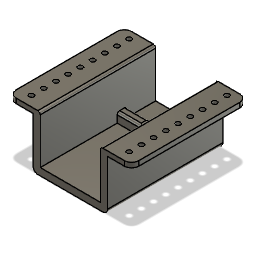
Motor mount (Autodesk Fusion 360 design; units mm, degrees)
Autodesk Fusion 360 part; units mm, degrees
sketch "Sketch1" plane through (0, 0, 0) normal (0, 1, 0) x (1, 0, 0)
  line L0 (0, 0) -> (12.5, 0)
  line L1 (12.5, 0) -> (12.5, 24)
  line L2 (12.5, 24) -> (0, 24)
  line L3 (0, 24) -> (0, 0)
  dimension "d1" = 12.5
  dimension "d2" = 24
  constraint horizontal L0
  constraint vertical L1
  constraint horizontal L2
  constraint vertical L3
  constraint coincident L0.start L3.end
  measures "d1" distance of L0.start L0.end
  measures "d2" distance of L0.start L2.end
extrude "Extrude1" add sketch "Sketch1" along normal blind 1.5
extrude "Extrude2" add 1 faces at (0, 0.5, -16) along direction (-1, 0, 0) blind 1.5
extrude "Extrude3" add 1 faces at (12.5, 0.5, -8) along direction (1, 0, 0) blind 1.5
sketch "Sketch2" plane through (0, 1.5, 0) normal (0, 1, 0) x (-1, 0, 0)
  line L0 (1.5, 0) -> (-14, 0)
  line L1 (-14, 0) -> (-14, -24)
  line L2 (-14, -24) -> (1.5, -24)
  line L3 (1.5, -24) -> (1.5, 0)
  line L4 (1.5, -24) -> (0, -24)
  line L5 (0, -24) -> (0, 0)
  line L6 (0, 0) -> (1.5, 0)
  line L7 (1.5, 0) -> (1.5, -24)
  line L8 (-14, -24) -> (-12.5, -24)
  line L9 (-12.5, -24) -> (-12.5, 0)
  line L10 (-12.5, 0) -> (-14, 0)
  line L11 (-14, 0) -> (-14, -24)
  dimension "d9" = 1.5
  constraint horizontal L4
  constraint vertical L5
  constraint horizontal L6
  constraint vertical L7
  constraint coincident L5.end L6.start
  constraint coincident L2.end L3.start
  constraint horizontal L8
  constraint vertical L9
  constraint horizontal L10
  constraint vertical L11
  constraint coincident L1.end L2.start
  measures "d9" distance of L1.end L8.end
extrude "Extrude4" add sketch "Sketch2" along normal blind 10 contours L0 L2 L3 L4 L5 L6 L7 | L0 L1 L2 L8 L9 L10 L11
sketch "Sketch3" plane through (14, 0, 0) normal (1, 0, 0) x (0, 0, -1)
  line L0 (0, 0) -> (24, 0)
  line L1 (24, 0) -> (24, 11.5)
  line L2 (24, 11.5) -> (0, 11.5)
  line L3 (0, 11.5) -> (0, 0)
  line L4 (0, 11.5) -> (24, 11.5)
  line L5 (24, 11.5) -> (24, 10.5)
  line L6 (24, 10.5) -> (0, 10.5)
  line L7 (0, 10.5) -> (0, 11.5)
  dimension "d12" = 1
  constraint horizontal L4
  constraint vertical L5
  constraint horizontal L6
  constraint vertical L7
  constraint coincident L2.end L3.start
  measures "d12" distance of L2.end L6.end
extrude "Extrude5" add sketch "Sketch3" along normal blind 5 contours L1 L2 L3 L4 L5 L6 L7
sketch "Sketch4" plane through (-1.5, 0, 0) normal (-1, 0, 0) x (0, 0, 1)
  line L0 (-24, 0) -> (0, 0)
  line L1 (0, 0) -> (0, 11.5)
  line L2 (0, 11.5) -> (-24, 11.5)
  line L3 (-24, 11.5) -> (-24, 0)
  line L4 (-24, 11.5) -> (0, 11.5)
  line L5 (0, 11.5) -> (0, 10.5)
  line L6 (0, 10.5) -> (-24, 10.5)
  line L7 (-24, 10.5) -> (-24, 11.5)
  dimension "d15" = 1
  constraint horizontal L4
  constraint vertical L5
  constraint horizontal L6
  constraint vertical L7
  constraint coincident L2.end L3.start
  measures "d15" distance of L2.end L6.end
extrude "Extrude6" add sketch "Sketch4" along normal blind 5 contours L1 L2 L3 L4 L5 L6 L7
ref_plane "WorkPlane1" through (-4, 10.5, -12) normal (0, -1, 0) x (0, 0, 1)
sketch "Sketch5" plane through (-4, 10.5, -12) normal (0, -1, 0) x (1, 0, 0)
  line L0 (23, 12) -> (23, -12)
  line L1 (-2.5, -12) -> (-2.5, 12)
  point P0 (0.09, 9.9032)
  point P1 (20.41, 9.9032)
  point P2 (0.09, 7.3632)
  point P3 (0.09, 4.8232)
  point P4 (0.09, 2.2832)
  point P5 (0.09, -0.2568)
  point P6 (0.09, -2.7968)
  point P7 (0.09, -5.3368)
  point P8 (0.09, -7.8768)
  point P9 (0.09, -10.4168)
  point P10 (20.41, 7.3632)
  point P11 (20.41, 4.8232)
  point P12 (20.41, 2.2832)
  point P13 (20.41, -0.2568)
  point P14 (20.41, -2.7968)
  point P15 (20.41, -5.3368)
  point P16 (20.41, -7.8768)
  point P17 (20.41, -10.4168)
  dimension "d19" = 20.32
  dimension "d20" = 2.59
  dimension "d21" = 2.59
  dimension "d24" = 0
  dimension "d25" = -20.32
  dimension "d28" = 0
  dimension "d29" = -20.32
  constraint horizontal P0 P1
  measures "d19" distance of P0 P1
  measures "d20" distance of P1 L0
  measures "d21" distance of P0 L1
hole "Hole1" at (-3.91, 10.5, -2.0968) at (-3.91, 10.5, -4.6368) at (-3.91, 10.5, -7.1768) at (-3.91, 10.5, -9.7168) at (-3.91, 10.5, -12.2568) at (-3.91, 10.5, -14.7968) at (-3.91, 10.5, -17.3368) at (-3.91, 10.5, -19.8768) at (-3.91, 10.5, -22.4168) at (16.41, 10.5, -2.0968) at (16.41, 10.5, -4.6368) at (16.41, 10.5, -7.1768) at (16.41, 10.5, -9.7168) at (16.41, 10.5, -12.2568) at (16.41, 10.5, -14.7968) at (16.41, 10.5, -17.3368) at (16.41, 10.5, -19.8768) at (16.41, 10.5, -22.4168) direction (0, 1, 0) diameter 1 depth 7 tip angle 118
sketch "Sketch6" plane through (0, 1.5, 0) normal (0, 1, 0) x (-1, 0, 0)
  line L0 (-12.5, 0) -> (-12.5, -24)
  line L1 (-12.5, -24) -> (0, -24)
  line L2 (0, -24) -> (0, 0)
  line L3 (0, 0) -> (-12.5, 0)
  line L4 (0, -18) -> (-5, -18)
  line L5 (-5, -18) -> (-5, -16)
  line L6 (-5, -16) -> (0, -16)
  line L7 (0, -16) -> (0, -18)
  dimension "d33" = 5
  dimension "d34" = 2
  dimension "d35" = 6
  constraint horizontal L4
  constraint vertical L5
  constraint horizontal L6
  constraint vertical L7
  constraint coincident L2 L4.start
  measures "d33" distance of L4.start L4.end
  measures "d34" distance of L4.start L6.end
  measures "d35" distance of L1 L4
extrude "Extrude7" add sketch "Sketch6" along normal blind 2 contours L2 L4 L5 L6 L7
fillet "Fillet1" radius 1 2 edges at (-1.5, 0, -12) (14, 0, -12)
fillet "Fillet2" radius 0.5 2 edges at (0, 11.5, -12) (12.5, 11.5, -12)
fillet "Fillet3" radius 1.5 4 edges at (19, 11, -24) (19, 11, 0) (-6.5, 11, 0) (-6.5, 11, -24)
fillet "Fillet4" radius 0.5 3 edges at (5, 3.5, -17) (2.5, 3.5, -18) (2.5, 3.5, -16)
